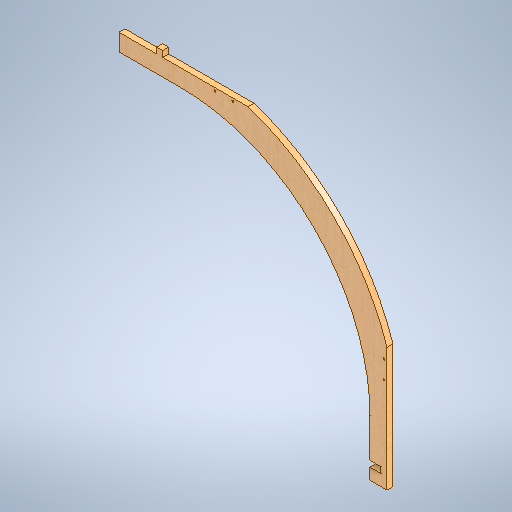
# Autodesk Inventor part: rail_test_90_nsoro
Saved by Autodesk Inventor 2025.1 (Build 291241000, 241)
## iProperties
Created: 2024-12-02
Part Number: rail_test_90_nsoro
Material: 一般
Document SubType Name: Modeling
Designer: yuki0520
Density: 1 g/cm^3
Appearance: イエロー パイン材 - 硬質 塗装 抑えた光沢
Author: yuki0520
Autodesk Inventor part; units mm, degrees
ref_plane "YZ Plane" through (0, 0, 0) normal (1, 0, 0) x (0, 1, 0)
ref_plane "XZ Plane" through (0, 0, 0) normal (0, 1, 0) x (-1, 0, 0)
ref_plane "XY Plane" through (0, 0, 0) normal (0, 0, 1) x (1, 0, 0)
derived "zzz_yoko3.ipt"
sketch "スケッチ1" plane through (0, 0, 0) normal (0, 0, 1) x (1, 0, 0)
  circle A0 centre (0, 0) radius 77
  line L0 (45, -80) -> (-45, -80)
  line L1 (-45, -80) -> (-45, 80)
  line L2 (-45, 80) -> (45, 80)
  line L3 (45, 80) -> (45, -80)
  line L4 (45, -80) -> (-45, 80) construction
  line L5 (-45, -80) -> (45, 80) construction
  circle A1 centre (197, 0) radius 120
  circle A2 centre (0, 197) radius 120
  line L6 (-45, 0) -> (45, 0)
  arc A3 (317, 0) -> (0, 317) centre (0, 0) ccw
  line L7 (0, 0) -> (0, 317) construction
  line L8 (0, 0) -> (317, 0) construction
  line L9 (0, 317) -> (0, 0)
  line L10 (317, 0) -> (0, 0)
  line L11 (335.5, -103) -> (317, -103)
  line L12 (317, -103) -> (317, 103)
  line L13 (317, 103) -> (335.5, 103)
  line L14 (335.5, 103) -> (335.5, -103)
  line L15 (335.5, -103) -> (317, 103) construction
  line L16 (317, -103) -> (335.5, 103) construction
  line L17 (-103, 317) -> (-103, 335.5)
  line L18 (-103, 335.5) -> (103, 335.5)
  line L19 (103, 335.5) -> (103, 317)
  line L20 (103, 317) -> (-103, 317)
  line L21 (-35, -80) -> (-35, 345.5)
  line L22 (0, 317) -> (0, 347)
  line L23 (317, 0) -> (347, 0)
  line L24 (227.3, -103) -> (166.7, -103)
  line L25 (166.7, -103) -> (166.7, 103)
  line L26 (166.7, 103) -> (227.3, 103)
  line L27 (227.3, 103) -> (227.3, -103)
  line L28 (227.3, -103) -> (166.7, 103) construction
  line L29 (166.7, -103) -> (227.3, 103) construction
  line L30 (197, 103) -> (197, -103)
  line L31 (-45, 94) -> (355, 94)
  line L32 (-45, -94) -> (355, -94)
  line L33 (35, -80) -> (35, 345.5)
  line L34 (-113, 335.5) -> (113, 335.5)
  line L35 (113, 335.5) -> (113, 345.5)
  line L36 (113, 345.5) -> (-113, 345.5)
  line L37 (-113, 345.5) -> (-113, 335.5)
  line L38 (35, 345.5) -> (45, 345.5)
  line L39 (45, 345.5) -> (45, 355.5)
  line L40 (45, 355.5) -> (35, 355.5)
  line L41 (35, 355.5) -> (35, 345.5)
  circle A4 centre (0, 0) radius 9
  line L42 (335.5, 113) -> (345.5, 113)
  line L43 (345.5, 113) -> (345.5, -107)
  line L44 (345.5, -107) -> (335.5, -107)
  line L45 (335.5, -107) -> (335.5, 113)
  arc A5 (345.5, 113) -> (113, 345.5) centre (0, 0) ccw
  line L46 (103, 335.5) -> (103, 299.7999)
  line L47 (335.5, 103) -> (299.7999, 103)
  line L48 (113, 345.5) -> (113, 296.1756)
  line L49 (-40, -80) -> (-30, -80)
  line L50 (-30, -80) -> (-30, 355.5)
  line L51 (-30, 355.5) -> (-40, 355.5)
  line L52 (-40, 345.5) -> (-40, -80)
  line L53 (-45, -75) -> (345.5, -75)
  line L54 (345.5, -75) -> (345.5, -65)
  line L55 (345.5, -65) -> (-45, -65)
  line L56 (-45, -65) -> (-45, -75)
  line L57 (-40, 345.5) -> (-50, 345.5)
  line L58 (-30, 355.5) -> (-40, 355.5)
  line L59 (-50, 345.5) -> (-40, 345.5)
  line L60 (-40, 345.5) -> (-40, 355.5)
  line L61 (-40, 355.5) -> (-50, 355.5)
  line L62 (-50, 355.5) -> (-50, 345.5)
  line L63 (-45, 80) -> (-55, 80)
  line L64 (-55, 80) -> (-55, 70)
  line L65 (-55, 70) -> (-45, 70)
  line L66 (-45, 70) -> (-45, 80)
  line L67 (-45, -80) -> (-55, -80)
  line L68 (75, -65) -> (75, -75)
  line L69 (-45, -80) -> (345.5, -80)
  line L70 (-45, -65) -> (-70, -65)
  line L71 (-70, -65) -> (-70, -75)
  line L72 (-70, -75) -> (-45, -75)
  line L73 (-45, -75) -> (-45, -65)
  line L74 (345.5, -75) -> (370.5, -75)
  line L75 (370.5, -75) -> (370.5, -65)
  line L76 (370.5, -65) -> (345.5, -65)
  line L77 (345.5, -65) -> (345.5, -75)
  line L78 (-103, 335.5) -> (-103, 345.5)
  point P0 (326.25, 0)
  point P1 (0, 335.5)
  point P2 (197, 0)
  point P3 (317, -65)
  point P4 (-40, 317)
  point P5 (0, 317)
  point P6 (317, -94)
  point P7 (345.5, -94)
  point P8 (335.5, -65)
  point P9 (335.5, -75)
  point P10 (317, -75)
  point P11 (-30, 345.5)
extrude "押し出し1" add sketch "スケッチ1" along normal blind 10 contours L23 L14 L55 L12 | A3 L31 L12 | L12 L31 L14 L23 | A3 L47 L12 L31 | L12 L13 L14 L31 | L23 L43 L55 L14 | L14 L31 L43 L23 | A3 L48 L35 A5 L42 L45 L13 L47 | L53 L14 L69 L12 | L55 L43 L53 L14 | L14 L45 L42 L43 L31 | A3 L46 L19 L34 L48 | L20 L33 A3 | L22 L18 L33 L20 | L20 L50 L18 L22 | L33 L20 L46 A3 | L69 L14 L32 L12 | L53 L43 L69 L14 | L34 L18 L33 L36 L35 | L33 L18 L19 L20 | L20 L21 L18 L50 | L22 L36 L33 L18 | L18 L50 L36 L22 | L69 L43 L32 L14 | L20 L52 L18 L21 | L18 L21 L36 L50 | L20 L17 L18 L52 | L18 L52 L36 L21 | L36 L60 L51 L50 | L18 L78 L36 L52
sketch "スケッチ2" plane through (-103, 345.5, 10) normal (0, 0, 1) x (1, 0, 0)
  line L0 (448.5, -439.5) -> (448.5, -232.5) projected
  arc A0 (448.5, -232.5) -> (216, 0) centre (103, -345.5) ccw projected
  line L1 (216, 0) -> (73, 0) projected
  line L2 (0, 0) -> (0, -28.5) projected
  line L3 (0, -28.5) -> (103, -28.5) projected
  arc A1 (420, -345.5) -> (103, -28.5) centre (103, -345.5) ccw projected
  line L4 (420, -345.5) -> (420, -410.5) projected
  line L5 (420, -439.5) -> (448.5, -439.5) projected
  line L6 (216, 0) -> (216, -49.3244)
  line L7 (0, -5) -> (216, -5)
  line L8 (448.5, -232.5) -> (399.1756, -232.5)
  arc A2 (420, -345.5) -> (103, -28.5) centre (103, -345.5) ccw projected
  line L9 (443.5, -439.5) -> (443.5, -232.5)
  line L10 (420, -410.5) -> (438.5, -410.5) projected
  line L11 (438.5, -410.5) -> (438.5, -420.5) projected
  line L12 (438.5, -420.5) -> (420, -420.5) projected
  line L13 (420, -420.5) -> (420, -439.5) projected
  line L14 (73, 0) -> (73, 10) projected
  line L15 (73, 10) -> (63, 10) projected
  line L16 (63, 10) -> (63, 0) projected
  line L17 (63, 0) -> (0, 0) projected
  point P0 (190.5, -5)
  point P1 (160.5, -5)
  point P2 (216, -24.6622)
  point P3 (443.5, -252)
  point P4 (443.5, -282)
  dimension "d4" = 30
  dimension "d6" = 30
  dimension "d14" = 5
  dimension "d15" = 5
  dimension "d16" = 187.5
  dimension "d17" = 190.5
  constraints: 8 end point, 6 point on line, 2 parallel, 2 perpendicular, 2 point on circle, 1 midpoint
  measures "d4" distance of point (160.5, -5) point (190.5, -5)
  measures "d6" distance of point (443.5, -282) point (443.5, -252)
  measures "d14" distance between parallel lines of L1 L7
  measures "d15" distance between parallel lines of L0 L9
  measures "d16" distance from line of L5 point (443.5, -252)
  measures "d17" distance from line of L2 point (190.5, -5)
hole "穴1" at (87.5, 340.5, 10) at (57.5, 340.5, 10) at (340.5, 93.5, 10) at (340.5, 63.5, 10) direction (0, 0, -1) diameter 3.2 end through all
